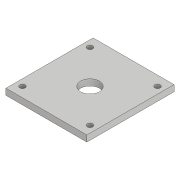
# Autodesk Inventor part: topPlate
Saved by Autodesk Inventor 2018.2 (Build 222227000, 227)
## iProperties
Created: 2018-05-06
Part Number: topPlate
Material: Generic
Document SubType Name: Modeling
Designer: sawaiz
Density: 1 g/cm^3
Appearance: Default
Author: sawaiz
Autodesk Inventor part; units mm, degrees
ref_plane "YZ Plane" through (0, 0, 0) normal (1, 0, 0) x (0, 1, 0)
ref_plane "XZ Plane" through (0, 0, 0) normal (0, 1, 0) x (-1, 0, 0)
ref_plane "XY Plane" through (0, 0, 0) normal (0, 0, 1) x (1, 0, 0)
sketch "Sketch1" plane through (0, 0, 0) normal (0, 1, 0) x (-1, 0, 0)
  line L0 (44.45, 41.275) -> (-44.45, 41.275)
  line L1 (-44.45, 41.275) -> (-44.45, -41.275)
  line L2 (-44.45, -41.275) -> (44.45, -41.275)
  line L3 (44.45, -41.275) -> (44.45, 41.275)
  line L4 (44.45, 41.275) -> (-44.45, -41.275) construction
  line L5 (-44.45, 41.275) -> (44.45, -41.275) construction
  point P0 (0, 0)
  dimension "d0" = 88.9
  dimension "d1" = 82.55
  constraints: 12 end point, 2 midpoint, 2 parallel, 1 horizontal, 1 perpendicular
  measures "d0" distance of L2.end L1.end
  measures "d1" distance of L1.end L0.end
extrude "Extrusion1" add sketch "Sketch1" along normal blind 6.35
sketch "Sketch2" plane through (0, 6.35, 0) normal (0, 1, 0) x (1, 0, 0)
  line L0 (34.45, -34.45) -> (-34.45, -34.45) construction
  line L1 (-34.45, -34.45) -> (-34.45, 34.45) construction
  line L2 (-34.45, 34.45) -> (34.45, 34.45) construction
  line L3 (34.45, 34.45) -> (34.45, -34.45) construction
  line L4 (34.45, -34.45) -> (-34.45, 34.45) construction
  line L5 (-34.45, -34.45) -> (34.45, 34.45) construction
  line L6 (-44.45, -41.275) -> (44.45, -41.275) projected
  line L7 (44.45, -41.275) -> (44.45, 41.275) projected
  line L8 (44.45, 41.275) -> (-44.45, 41.275) projected
  line L9 (-44.45, 41.275) -> (-44.45, -41.275) projected
  point P0 (0, 0)
  dimension "d4" = 68.9
  dimension "d5" = 68.9
  dimension "d20" = 88.9
  constraints: 12 end point, 4 coincident, 2 midpoint, 2 parallel, 1 horizontal, 1 perpendicular
  measures "d4" distance of L1.end L2.end
  measures "d5" distance of L0.end L1.end
  measures "d20" distance of L7.end L8.end
hole "Hole1" at (-34.45, 6.35, 34.45) at (-34.45, 6.35, -34.45) at (34.45, 6.35, -34.45) at (34.45, 6.35, 34.45) direction (0, -1, 0) diameter 5.5 depth 8 tip angle 118 clearance for "Hex Head Bolt" size "M5" standard "Ansi Metric M Profile"
sketch "Sketch3" plane through (0, 6.35, 0) normal (0, 1, 0) x (1, 0, 0)
  point P0 (0, 0)
  point P1 (0, 0)
  constraints: 1 coincident
hole "Hole2" at (0, 6.35, 0) direction (0, -1, 0) diameter 19.05 end through all
equation "\"d5\" = d4"
body "Solid1"
